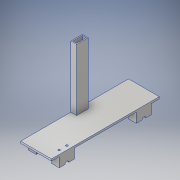
# Autodesk Inventor part: longSupportPlateV02
Saved by Autodesk Inventor 2016 SP1 (Build 200210100, 210)
## iProperties
Created: 2016-02-05
Part Number: longSupportPlateV02
Material: Aluminum 6061
Document SubType Name: Modeling
Designer: steele
Density: 2.7 g/cm^3
Appearance: Aluminum - Flat
Mass: 707.921 g
Surface Area: 890.321 cm^2
Volume: 262.193 cm^3
Author: steele
Autodesk Inventor part; units mm, degrees
ref_plane "YZ Plane" through (0, 0, 0) normal (1, 0, 0) x (0, 1, 0)
ref_plane "XZ Plane" through (0, 0, 0) normal (0, 1, 0) x (-1, 0, 0)
ref_plane "XY Plane" through (0, 0, 0) normal (0, 0, 1) x (1, 0, 0)
sketch "Sketch1" plane through (0, 0, 0) normal (0, 1, 0) x (-1, 0, 0)
  line L0 (50.8, 177.8) -> (-50.8, 177.8)
  line L1 (-50.8, 177.8) -> (-50.8, -177.8)
  line L2 (-50.8, -177.8) -> (50.8, -177.8)
  line L3 (50.8, -177.8) -> (50.8, 177.8)
  line L4 (50.8, 177.8) -> (-50.8, -177.8) construction
  line L5 (-50.8, 177.8) -> (50.8, -177.8) construction
  point P0 (0, 0)
  dimension "d0" = 355.6
  dimension "d1" = 101.6
  constraints: 12 end point, 2 midpoint, 2 parallel, 1 horizontal, 1 perpendicular
  measures "d0" distance of L2.end L0.start
  measures "d1" distance of L0.start L0.end
extrude "Extrusion1" add sketch "Sketch1" along normal blind 6.35
sketch "Sketch4" plane through (0, 0, 0) normal (0, -1, 0) x (1, 0, 0)
  line L0 (-50.8, -177.8) -> (-50.8, 177.8) projected
  line L1 (-50.8, 101.6) -> (-25.4, 101.6)
  line L2 (-25.4, 101.6) -> (-25.4, 152.4)
  line L3 (-25.4, 152.4) -> (-50.8, 152.4)
  line L4 (-50.8, 152.4) -> (-50.8, 101.6)
  line L5 (-50.8, 177.8) -> (50.8, 177.8) projected
  point P0 (0, 0)
  dimension "d15" = 25.4
  dimension "d16" = 50.8
  dimension "d17" = 25.4
  constraints: 8 end point, 2 parallel, 1 horizontal, 1 perpendicular, 1 point on line
  measures "d15" distance of L2.end L3.end
  measures "d16" distance of L1.end L2.end
  measures "d17" distance between parallel lines of L5 L3
extrude "Extrusion4" add sketch "Sketch4" along normal blind 31.75
sketch "Sketch6" plane through (-50.8, 6.35, -177.8) normal (-1, 0, 0) x (0, 0, 1)
  line L0 (330.2, -38.1) -> (279.4, -38.1) projected
  circle A0 centre (304.8, -38.1) radius 6.35
  point P0 (177.8, -6.35)
  dimension "d21" = 12.7
  constraints: 1 centre point, 1 midpoint
  measures "d21" diameter of A0
extrude "Extrusion5" cut sketch "Sketch6" against normal through all
mirror "Mirror1" about plane through (0, 0, 0) normal (1, 0, 0) of "Extrusion4", "Extrusion5"
sketch "Sketch7" plane through (0, 0, 0) normal (0, -1, 0) x (1, 0, 0)
  line L0 (50.8, 177.8) -> (50.8, -177.8) projected
  line L1 (50.8, -101.6) -> (25.4, -101.6)
  line L2 (25.4, -101.6) -> (25.4, -152.4)
  line L3 (25.4, -152.4) -> (50.8, -152.4)
  line L4 (50.8, -152.4) -> (50.8, -101.6)
  line L5 (-50.8, 177.8) -> (50.8, 177.8) projected
  point P0 (0, 0)
  dimension "d24" = 279.4
  dimension "d25" = 50.8
  dimension "d26" = 25.4
  constraints: 8 end point, 2 parallel, 1 horizontal, 1 perpendicular, 1 point on line
  measures "d24" distance between parallel lines of L1 L5
  measures "d25" distance of L1.end L2.end
  measures "d26" distance of L2.end L3.end
extrude "Extrusion6" add sketch "Sketch7" along normal blind 31.75
sketch "Sketch8" plane through (50.8, 6.35, 177.8) normal (1, 0, 0) x (0, 0, -1)
  line L0 (279.4, -38.1) -> (330.2, -38.1) projected
  circle A0 centre (304.8, -38.1) radius 6.35
  point P0 (177.8, -6.35)
  dimension "d29" = 12.7
  constraints: 1 centre point, 1 midpoint
  measures "d29" diameter of A0
extrude "Extrusion7" cut sketch "Sketch8" against normal through all
mirror "Mirror2" about plane through (0, 0, 0) normal (1, 0, 0) of "Extrusion6", "Extrusion7"
sketch "Sketch9" plane through (0, 6.35, 0) normal (0, 1, 0) x (1, 0, 0)
  point P0 (38.1, -114.3)
  point P1 (38.1, -139.7)
hole "Hole1" at (38.1, 6.35, 114.3) at (38.1, 6.35, 139.7) direction (0, -1, 0) diameter 6.7564 depth 38.1
sketch "Sketch14" plane through (0, 6.35, 0) normal (0, 1, 0) x (1, 0, 0)
  line L0 (-31.75, -12.2936) -> (-31.75, 25.8064)
  line L1 (-31.75, 25.8064) -> (-50.8, 25.8064)
  line L2 (-50.8, 25.8064) -> (-50.8, -12.2936)
  line L3 (-50.8, -12.2936) -> (-31.75, -12.2936)
  line L4 (-31.75, -12.2936) -> (-50.8, 25.8064) construction
  line L5 (-31.75, 25.8064) -> (-50.8, -12.2936) construction
  line L6 (50.8, 177.8) -> (-50.8, 177.8) projected
  line L7 (-50.8, 177.8) -> (-50.8, -177.8) projected
  line L8 (-34.925, -9.1186) -> (-34.925, 22.6314)
  line L9 (-34.925, 22.6314) -> (-47.625, 22.6314)
  line L10 (-47.625, 22.6314) -> (-47.625, -9.1186)
  line L11 (-47.625, -9.1186) -> (-34.925, -9.1186)
  line L12 (-34.925, -9.1186) -> (-47.625, 22.6314) construction
  line L13 (-34.925, 22.6314) -> (-47.625, -9.1186) construction
  point P0 (0, 0)
  point P1 (-41.275, 6.7564)
  dimension "d49" = 171.0436
  dimension "d50" = 19.05
  dimension "d51" = 38.1
  dimension "d52" = 3.175
  dimension "d53" = 3.175
  constraints: 24 end point, 4 midpoint, 4 parallel, 2 perpendicular, 2 vertical, 1 collinear
  measures "d49" distance from line of point (-41.275, 6.756) L6
  measures "d50" distance of L2.end L0.start
  measures "d51" distance of L0.start L0.end
  measures "d52" distance between parallel lines of L10 L2
  measures "d53" distance between parallel lines of L3 L11
extrude "Extrusion10" add sketch "Sketch14" along normal blind 203.2
equation "\"d0\" = plateLength"
equation "\"d1\" = plateWidth"
equation "\"d2\" = plateThickness"
equation "\"d18\" = extensionSupportLength"
equation "\"d27\" = extensionSupportLength"
equation "\"d49\" = distanceFromRearToCenterOfMiddleSprocket"
equation "\"d50\" = widthOfCenterPost"
equation "\"d51\" = lengthOfCenterPost"
equation "\"d52\" = wallWidthOfCenterPost"
equation "\"d53\" = wallWidthOfCenterPost"
equation "\"d54\" = heightOfCenterPost"
equation "\"plateWidth\" = 101.6"
equation "\"plateLength\" = 355.6"
equation "\"plateThickness\" = 6.35"
equation "\"extensionSupportLength\" = 31.75"
equation "\"distanceFromRearToCenterOfMiddleSprocket\" = 171.0436"
equation "\"widthOfCenterPost\" = 19.05"
equation "\"lengthOfCenterPost\" = 38.1"
equation "\"wallWidthOfCenterPost\" = 3.175"
equation "\"heightOfCenterPost\" = 203.2"
body "Solid1"
